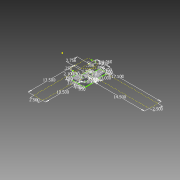
# Autodesk Inventor part: Laser_Holder
Saved by Autodesk Inventor 2013 (Build 170138000, 138)
## iProperties
Created: 2015-03-30
Part Number: Laser_Holder
Material: Generic
Document SubType Name: Modeling
Designer: Pat
Density: 1 g/cm^3
Author: Pat
Autodesk Inventor part; units mm, degrees
ref_plane "YZ Plane" through (0, 0, 0) normal (1, 0, 0) x (0, 1, 0)
ref_plane "XZ Plane" through (0, 0, 0) normal (0, 1, 0) x (-1, 0, 0)
ref_plane "XY Plane" through (0, 0, 0) normal (0, 0, 1) x (1, 0, 0)
sketch "Sketch1" plane through (0, 0, 0) normal (0, 1, 0) x (-1, 0, 0)
  line L0 (-203.3861, 74.2822) -> (-125.9161, 74.2822) construction
  line L1 (-125.9161, 74.2822) -> (-125.9161, -61.6078) construction
  line L2 (-125.9161, -61.6078) -> (-203.3861, -61.6078) construction
  line L3 (-203.3861, -61.6078) -> (-203.3861, 74.2822) construction
  line L4 (-203.3861, 74.2822) -> (-266.8861, 74.2822) construction
  line L5 (-164.6511, 373.4543) -> (-228.1511, 373.4543) construction
  line L6 (-228.1511, 373.4543) -> (-228.1511, 106.7543) construction
  line L7 (-228.1511, 106.7543) -> (-299.9932, 34.9122) construction
  line L8 (-299.9932, 34.9122) -> (-668.2932, 34.9122) construction
  line L9 (-668.2932, 34.9122) -> (-668.2932, -28.5878) construction
  line L10 (-668.2932, -28.5878) -> (-223.7932, -28.5878) construction
  line L11 (-223.7932, -28.5878) -> (-164.6511, 30.5543) construction
  line L12 (-164.6511, 30.5543) -> (-164.6511, 373.4543) construction
  line L13 (-264.0722, 70.8332) -> (-194.2222, 0.9832) construction
  line L14 (-266.8861, 74.2822) -> (-266.8861, 48.8822) construction
  line L15 (-266.8861, 48.8822) -> (-203.3861, -14.6178) construction
  line L16 (-266.8861, 68.0193) -> (-260.6232, 74.2822) construction
  circle A0 centre (-251.4998, 58.2609) radius 2.54
  circle A1 centre (-215.5788, 22.3399) radius 2.54
  line L17 (-264.6511, 135.2422) -> (-188.4511, 135.2422)
  line L18 (-188.4511, 135.2422) -> (-188.4511, 81.9022)
  line L19 (-188.4511, 81.9022) -> (-264.6511, 81.9022)
  line L20 (-264.6511, 81.9022) -> (-264.6511, 135.2422)
  circle A2 centre (-164.6511, -28.5878) radius 4.9213 construction
  line L21 (-164.6511, 30.5543) -> (-164.6511, -28.5878) construction
  line L22 (-164.6511, -28.5878) -> (-223.7932, -28.5878) construction
  line L23 (-264.6511, 136.5122) -> (-187.1811, 136.5122)
  line L24 (-187.1811, 136.5122) -> (-187.1811, 80.6322)
  line L25 (-187.1811, 80.6322) -> (-264.6511, 80.6322)
  line L26 (-264.6511, 80.6322) -> (-264.6511, 136.5122)
  line L27 (-289.7461, 41.4122) -> (-236.4061, 41.4122)
  line L28 (-236.4061, 41.4122) -> (-236.4061, -34.7878)
  line L29 (-236.4061, -34.7878) -> (-289.7461, -34.7878)
  line L30 (-289.7461, -34.7878) -> (-289.7461, 41.4122)
  line L31 (-291.0161, 42.6822) -> (-235.1361, 42.6822)
  line L32 (-235.1361, 42.6822) -> (-235.1361, -36.0578)
  line L33 (-235.1361, -36.0578) -> (-291.0161, -36.0578)
  line L34 (-291.0161, -36.0578) -> (-291.0161, 42.6822)
  line L35 (-235.1361, -5.4793) -> (-209.7361, 19.9207)
  line L36 (-209.7361, 19.9207) -> (-209.7361, 80.6322)
  line L37 (-264.6511, 136.5122) -> (-264.6511, 80.6322)
  line L38 (-264.6511, 81.9022) -> (-264.6511, 135.2422)
  line L39 (-264.6511, 80.6322) -> (-264.6511, 136.5122)
  line L40 (-265.9211, 135.2422) -> (-297.6711, 135.2422)
  line L41 (-297.6711, 135.2422) -> (-297.6711, 81.9022)
  line L42 (-297.6711, 81.9022) -> (-265.9211, 81.9022)
  line L43 (-265.9211, 81.9022) -> (-265.9211, 135.2422)
  line L44 (-264.6511, 136.5122) -> (-298.9411, 136.5122)
  line L45 (-298.9411, 136.5122) -> (-298.9411, 80.6322)
  line L46 (-298.9411, 80.6322) -> (-264.6511, 80.6322)
  line L47 (-291.0161, 42.6822) -> (-298.9411, 80.6322)
  point P0 (0, 0)
  point P1 (-177.3511, 74.2822)
  point P2 (-151.9511, 74.2822)
  point P3 (-177.3511, -61.6078)
  point P4 (-151.9511, -61.6078)
  dimension "d0" = 63.5
  dimension "d1" = 63.5
  dimension "d2" = 63.5
  dimension "d3" = 101.6
  dimension "d4" = 266.7
  dimension "d5" = 368.3
  dimension "d6" = 444.5
  dimension "d7" = 342.9
  dimension "d8" = 17.78
  dimension "d9" = 68.58
  dimension "d10" = 25.4
  dimension "d11" = 5.08
  dimension "d12" = 5.08
  dimension "d14" = 76.2
  dimension "d15" = 9.8425
  dimension "d16" = 59.142
  dimension "d17" = 100
  dimension "d20" = 1.27
  dimension "d22" = 6.35
  dimension "d26" = 53.34
  dimension "d27" = 1.27
  dimension "d28" = 1.27
  dimension "d29" = 1.27
  dimension "d30" = 1.27
  dimension "d31" = 76.2
  dimension "d32" = 31.75
  dimension "d33" = 70
  dimension "d42" = 6.35
  dimension "d43" = 5.8426
  dimension "d44" = 5.842
  dimension "d50" = 31.75
  dimension "d51" = 1.27
  dimension "d52" = 1.27
  dimension "d53" = 53.34
  dimension "d54" = 1.27
  dimension "d55" = 1.27
  constraints: 97 end point, 19 parallel, 16 point on line, 15 perpendicular, 6 horizontal, 4 collinear, 3 centre point, 2 midpoint, 1 coincident
  measures "d0" distance of L4.start L4.end
  measures "d1" distance of L5.start L6.start
  measures "d2" distance of L9.start L10.start
  measures "d3" distance of L6.end L8.start
  measures "d4" distance of L6.start L6.end
  measures "d5" distance of L8.start L9.start
  measures "d6" distance of L11.start L10.start
  measures "d7" distance of L12.start L5.start
  measures "d8" distance from line of L7 point (-251.5, 58.261)
  measures "d9" distance from line of L7 point (-215.579, 22.34)
  measures "d10" distance of L4.end L15.start
  measures "d11" diameter of A0
  measures "d12" diameter of A1
  measures "d14" distance of L17.start L17.end
  measures "d15" diameter of A2
  measures "d16" distance of L11.start A2.centre
  measures "d17" distance from line of L22.start L20
  measures "d20" distance between parallel lines of L24 L18
  measures "d22" distance between parallel lines of L25 L0
  measures "d26" distance of L28.end L29.end
  measures "d27" distance between parallel lines of L32 L28
  measures "d28" distance between parallel lines of L30 L34
  measures "d29" distance between parallel lines of L33 L29
  measures "d30" distance between parallel lines of L31 L27
  measures "d31" distance between parallel lines of L29 L27
  measures "d32" distance between parallel lines of L3 L32
  measures "d33" distance from line of L27 A2.centre
  measures "d42" distance between parallel lines of L3 L36
  measures "d43" distance from line of L36 A1.centre
  measures "d44" distance from line of L35 point (-215.579, 22.34)
  measures "d50" distance of L40.start L40.end
  measures "d51" distance between parallel lines of L19 L25
  measures "d52" distance between parallel lines of L23 L17
  measures "d53" distance between parallel lines of L19 L17
  measures "d54" distance between parallel lines of L39 L43
  measures "d55" distance between parallel lines of L45 L41
extrude "Extrusion6" add sketch "Sketch1" along normal blind 1.27 contours L26 L23 L24 L25 L19 L18 L17 | L17 L18 L19 L20 | L20 L26 L46 L45 L44 | L25 L36 L35 L32 L31 L47 L46 | L31 L32 L33 L34 | L27 L28 L29 L30 | L43 L42 L41 L40
extrude "Extrusion7" add sketch "Sketch1" along normal blind 12.7 contours L26 L23 L24 L25 L19 L18 L17
extrude "Extrusion8" add sketch "Sketch1" along normal blind 12.7 contours L31 L32 L33 L34
extrude "Extrusion9" add sketch "Sketch1" along normal blind 25.4 contours L20 L26 L46 L45 L44
sketch "Sketch6" plane through (0, 12.7, 0) normal (0, 1, 0) x (1, 0, 0)
  line L0 (187.1811, -80.6322) -> (187.1811, -136.5122) projected
  line L1 (188.4511, -81.9022) -> (187.1811, -81.9022)
  line L2 (187.1811, -81.9022) -> (187.1811, -135.2422)
  line L3 (187.1811, -135.2422) -> (188.4511, -135.2422)
  line L4 (188.4511, -135.2422) -> (188.4511, -81.9022)
  point P0 (0, 0)
  constraints: 8 end point, 2 parallel, 1 horizontal, 1 perpendicular, 1 point on line
extrude "Extrusion11" cut sketch "Sketch6" against normal blind 11.43
sketch "Sketch7" plane through (0, 12.7, 0) normal (0, 1, 0) x (1, 0, 0)
  line L0 (291.0161, 36.0578) -> (235.1361, 36.0578) projected
  line L1 (236.4061, 34.7878) -> (289.7461, 34.7878)
  line L2 (289.7461, 34.7878) -> (289.7461, 36.0578)
  line L3 (289.7461, 36.0578) -> (236.4061, 36.0578)
  line L4 (236.4061, 36.0578) -> (236.4061, 34.7878)
  point P0 (0, 0)
  constraints: 8 end point, 2 parallel, 1 horizontal, 1 perpendicular, 1 point on line
extrude "Extrusion12" cut sketch "Sketch7" against normal blind 11.43
body "Solid3"
